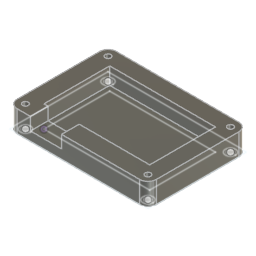
BottomPartVibePad (Autodesk Fusion 360 design; units mm, degrees)
Autodesk Fusion 360 part; units mm, degrees
sketch "Esboço1" plane through (0, 0, 0) normal (0, 0, 1) x (1, 0, 0) in component "VibePad Gaming"
  line L0 (0, 0) -> (62.9, 0)
  line L1 (62.9, 0) -> (62.9, 39.1)
  line L2 (62.9, 39.1) -> (0, 39.1)
  line L3 (0, 39.1) -> (0, 0)
  line L4 (-10.5, -10.5) -> (72.4, -10.5)
  line L5 (72.4, -10.5) -> (72.4, 48.6)
  line L6 (72.4, 48.6) -> (-10.5, 48.6)
  line L7 (-10.5, 48.6) -> (-10.5, -10.5)
  circle A0 centre (-5.5, 43.6) radius 1.7
  circle A1 centre (67.4, 43.6) radius 1.7
  circle A2 centre (67.4, -5.5) radius 1.7
  circle A3 centre (-5.5, -5.5) radius 1.7
  circle A4 centre (67.4, -5.5) radius 3
  circle A5 centre (67.4, 43.6) radius 3
  circle A6 centre (-5.5, 43.6) radius 3
  circle A7 centre (-5.5, -5.5) radius 3
  dimension "d1" = 62.9
  dimension "d2" = 39.1
  dimension "d3" = 82.9
  dimension "d4" = 59.1
  dimension "d5" = 9.5
  dimension "d6" = 9.5
  dimension "d7" = 3.4
  dimension "d8" = 3.4
  dimension "d9" = 3.4
  dimension "d10" = 3.4
  dimension "d11" = 5
  dimension "d12" = 5
  dimension "d13" = 5
  dimension "d14" = 5
  dimension "d15" = 5
  dimension "d16" = 5
  dimension "d17" = 5
  dimension "d18" = 5
  dimension "d19" = 6
  dimension "d20" = 6
  dimension "d21" = 6
  dimension "d22" = 6
  constraint horizontal L0
  constraint vertical L1
  constraint horizontal L2
  constraint vertical L3
  constraint coincident L0.start L3.end
  constraint horizontal L4
  constraint vertical L5
  constraint horizontal L6
  constraint vertical L7
  constraint concentric A2 A4
  constraint concentric A1 A5
  constraint concentric A0 A6
  constraint concentric A3 A7
  measures "d1" distance of L0.start L0.end
  measures "d2" distance of L0.start L2.end
  measures "d3" distance of L4.start L4.end
  measures "d4" distance of L4.start L6.end
  measures "d5" distance of L2 L6
  measures "d6" distance of L1 L5
  measures "d7" diameter of A0
  measures "d8" diameter of A1
  measures "d9" diameter of A2
  measures "d10" diameter of A3
  measures "d11" distance of L4 A3.centre
  measures "d12" distance of L7 A3.centre
  measures "d13" distance of L4 A2.centre
  measures "d14" distance of L5 A2.centre
  measures "d15" distance of L5 A1.centre
  measures "d16" distance of L6 A1.centre
  measures "d17" distance of L6 A0.centre
  measures "d18" distance of L7 A0.centre
  measures "d19" diameter of A4
  measures "d20" diameter of A5
  measures "d21" diameter of A6
  measures "d22" diameter of A7
extrude "Extrusão1" add sketch "Esboço1" along normal blind 9.9 from surface at 3.1 contours A4 | A5 | A6 | A7 makes body 1 at (66.0314, 40.9304, 6.4) makes body 2 at (-2.5037, 43.4505, 9.7) makes body 3 at (66.0314, -8.1696, 6.4) makes body 4 at (-2.5037, -5.6495, 9.7) in component "VibePad Gaming"
extrude "Extrusão2" add sketch "Esboço1" along normal blind 13 contours L4 L5 L6 L7 bodies 1 2 3 4 in component "VibePad Gaming"
extrude "Extrusão3" add sketch "Esboço1" along normal blind 3 contours L0 L1 L2 L3 bodies 1 in component "VibePad Gaming"
sketch "Esboço2" plane through (0, 0, 13) normal (0, 0, 1) x (-1, 0, 0) in component "VibePad Gaming"
  circle A0 centre (-67.4, -43.6) radius 1.7
  circle A1 centre (5.5, 5.5) radius 1.7
  line L0 (0, 0) -> (0, -39.1)
  line L1 (0, -39.1) -> (-62.9, -39.1)
  line L2 (-62.9, -39.1) -> (-62.9, 0)
  line L3 (-62.9, 0) -> (0, 0)
  line L4 (10.5, -48.6) -> (10.5, 10.5)
  line L5 (10.5, 10.5) -> (-72.4, 10.5)
  line L6 (-72.4, 10.5) -> (-72.4, -48.6)
  line L7 (-72.4, -48.6) -> (10.5, -48.6)
  circle A2 centre (5.5, -43.6) radius 1.7
  circle A3 centre (-67.4, 5.5) radius 1.7
  line L8 (-20.95, 0) -> (-2.45, 0)
  line L9 (-2.45, 0) -> (-2.45, 10.5)
  line L10 (-2.45, 10.5) -> (-20.95, 10.5)
  line L11 (-20.95, 10.5) -> (-20.95, 0)
  line L12 (10.5, -48.6) -> (10.5, 10.5)
  dimension "d30" = 18.5
  dimension "d31" = 12.95
  constraint horizontal L8
  constraint vertical L9
  constraint horizontal L10
  constraint vertical L11
  constraint coincident L5 L9.end
  constraint coincident L3 L8.start
  measures "d30" distance of L9 L11
  measures "d31" distance of L9 L12
extrude "Extrusão4" cut sketch "Esboço2" against normal blind 7.5 contours L3 L5 L8 L9 L10 L11 bodies 1 in component "VibePad Gaming"
fillet "Arredondamento1" radius 5 1 edges at (-10.5, 48.6, 6.5) on bodies 1 in component "VibePad Gaming"
fillet "Arredondamento2" radius 5 1 edges at (-10.5, -10.5, 6.5) on bodies 1 in component "VibePad Gaming"
fillet "Arredondamento3" radius 5 2 edges at (72.4, 48.6, 6.5) (72.4, -10.5, 6.5) on bodies 1 in component "VibePad Gaming"
component "VibePad Gaming" placed x (1, 0, 0) y (0, 1, 0) z (0, 0, 1) at (0, 0, 0)
